Autodesk Fusion 360 part; units mm, degrees
(part 2 of 6)
sketch "Sketch3" plane through (0, 0, 0) normal (0, 1, 0) x (-1, 0, 0)
  line L0 (-39.9203, -22.8327) -> (-39.9203, -25.9319)
  line L1 (-39.9203, -25.9319) -> (-40.7211, -25.9319)
  line L2 (-40.7211, -25.9319) -> (-40.7211, -31.7321)
  line L3 (-40.7211, -31.7321) -> (-39.9203, -31.7321)
  line L4 (-39.9203, -31.7321) -> (-39.9203, -34.8327)
  line L5 (-39.9203, -34.8327) -> (-40.7211, -34.8327)
  line L6 (-40.7211, -34.8327) -> (-40.7211, -35.8316)
  line L7 (-40.7211, -35.8316) -> (-54.7204, -35.8316)
  line L8 (-54.7204, -35.8316) -> (-54.7204, -34.8327)
  line L9 (-54.7204, -34.8327) -> (-55.5212, -34.8327)
  line L10 (-55.5212, -34.8327) -> (-55.5212, -31.7321)
  line L11 (-55.5212, -31.7321) -> (-54.7204, -31.7321)
  line L12 (-54.7204, -31.7321) -> (-54.7204, -25.9319)
  line L13 (-54.7204, -25.9319) -> (-55.5212, -25.9319)
  line L14 (-55.5212, -25.9319) -> (-55.5212, -22.8327)
  line L15 (-55.5212, -22.8327) -> (-54.7204, -22.8327)
  line L16 (-54.7204, -22.8327) -> (-54.7204, -21.8323)
  line L17 (-54.7204, -21.8323) -> (-40.7211, -21.8323)
  line L18 (-40.7211, -21.8323) -> (-40.7211, -22.8327)
  line L19 (-40.7211, -22.8327) -> (-39.9203, -22.8327)
  line L20 (-111.869, -35.8316) -> (-111.869, -34.8327)
  line L21 (-111.869, -34.8327) -> (-112.67, -34.8327)
  line L22 (-112.67, -34.8327) -> (-112.67, -31.7321)
  line L23 (-112.67, -31.7321) -> (-111.869, -31.7321)
  line L24 (-111.869, -31.7321) -> (-111.869, -25.9319)
  line L25 (-111.869, -25.9319) -> (-112.67, -25.9319)
  line L26 (-112.67, -25.9319) -> (-112.67, -22.8327)
  line L27 (-112.67, -22.8327) -> (-111.869, -22.8327)
  line L28 (-111.869, -22.8327) -> (-111.869, -21.8323)
  line L29 (-111.869, -21.8323) -> (-97.8697, -21.8323)
  line L30 (-97.8697, -21.8323) -> (-97.8697, -22.8327)
  line L31 (-97.8697, -22.8327) -> (-97.0703, -22.8327)
  line L32 (-97.0703, -22.8327) -> (-97.0703, -25.9319)
  line L33 (-97.0703, -25.9319) -> (-97.8697, -25.9319)
  line L34 (-97.8697, -25.9319) -> (-97.8697, -31.7321)
  line L35 (-97.8697, -31.7321) -> (-97.0703, -31.7321)
  line L36 (-97.0703, -31.7321) -> (-97.0703, -34.8327)
  line L37 (-97.0703, -34.8327) -> (-97.8697, -34.8327)
  line L38 (-97.8697, -34.8327) -> (-97.8697, -35.8316)
  line L39 (-97.8697, -35.8316) -> (-111.869, -35.8316)
  line L40 (-78.8211, -34.8327) -> (-78.8211, -35.8316)
  line L41 (-78.8211, -35.8316) -> (-92.8204, -35.8316)
  line L42 (-92.8204, -35.8316) -> (-92.8204, -34.8327)
  line L43 (-92.8204, -34.8327) -> (-93.6198, -34.8327)
  line L44 (-93.6198, -34.8327) -> (-93.6198, -31.7321)
  line L45 (-93.6198, -31.7321) -> (-92.8204, -31.7321)
  line L46 (-92.8204, -31.7321) -> (-92.8204, -25.9319)
  line L47 (-92.8204, -25.9319) -> (-93.6198, -25.9319)
  line L48 (-93.6198, -25.9319) -> (-93.6198, -22.8327)
  line L49 (-93.6198, -22.8327) -> (-92.8204, -22.8327)
  line L50 (-92.8204, -22.8327) -> (-92.8204, -21.8323)
  line L51 (-92.8204, -21.8323) -> (-78.8211, -21.8323)
  line L52 (-78.8211, -21.8323) -> (-78.8211, -22.8327)
  line L53 (-78.8211, -22.8327) -> (-78.0203, -22.8327)
  line L54 (-78.0203, -22.8327) -> (-78.0203, -25.9319)
  line L55 (-78.0203, -25.9319) -> (-78.8211, -25.9319)
  line L56 (-78.8211, -25.9319) -> (-78.8211, -31.7321)
  line L57 (-78.8211, -31.7321) -> (-78.0203, -31.7321)
  line L58 (-78.0203, -31.7321) -> (-78.0203, -34.8327)
  line L59 (-78.0203, -34.8327) -> (-78.8211, -34.8327)
  line L60 (-59.7711, -34.8327) -> (-59.7711, -35.8316)
  line L61 (-59.7711, -35.8316) -> (-73.7704, -35.8316)
  line L62 (-73.7704, -35.8316) -> (-73.7704, -34.8327)
  line L63 (-73.7704, -34.8327) -> (-74.5712, -34.8327)
  line L64 (-74.5712, -34.8327) -> (-74.5712, -31.7321)
  line L65 (-74.5712, -31.7321) -> (-73.7704, -31.7321)
  line L66 (-73.7704, -31.7321) -> (-73.7704, -25.9319)
  line L67 (-73.7704, -25.9319) -> (-74.5712, -25.9319)
  line L68 (-74.5712, -25.9319) -> (-74.5712, -22.8327)
  line L69 (-74.5712, -22.8327) -> (-73.7704, -22.8327)
  line L70 (-73.7704, -22.8327) -> (-73.7704, -21.8323)
  line L71 (-73.7704, -21.8323) -> (-59.7711, -21.8323)
  line L72 (-59.7711, -21.8323) -> (-59.7711, -22.8327)
  line L73 (-59.7711, -22.8327) -> (-58.9703, -22.8327)
  line L74 (-58.9703, -22.8327) -> (-58.9703, -25.9319)
  line L75 (-58.9703, -25.9319) -> (-59.7711, -25.9319)
  line L76 (-59.7711, -25.9319) -> (-59.7711, -31.7321)
  line L77 (-59.7711, -31.7321) -> (-58.9703, -31.7321)
  line L78 (-58.9703, -31.7321) -> (-58.9703, -34.8327)
  line L79 (-58.9703, -34.8327) -> (-59.7711, -34.8327)
  line L80 (-188.871, -41.8828) -> (-188.07, -41.8828)
  line L81 (-188.07, -41.8828) -> (-188.07, -40.8824)
  line L82 (-188.07, -40.8824) -> (-174.071, -40.8824)
  line L83 (-174.071, -40.8824) -> (-174.071, -41.8828)
  line L84 (-174.071, -41.8828) -> (-173.27, -41.8828)
  line L85 (-173.27, -41.8828) -> (-173.27, -44.982)
  line L86 (-173.27, -44.982) -> (-174.071, -44.982)
  line L87 (-174.071, -44.982) -> (-174.071, -50.782)
  line L88 (-174.071, -50.782) -> (-173.27, -50.782)
  line L89 (-173.27, -50.782) -> (-173.27, -53.8826)
  line L90 (-173.27, -53.8826) -> (-174.071, -53.8826)
  line L91 (-174.071, -53.8826) -> (-174.071, -54.8816)
  line L92 (-174.071, -54.8816) -> (-188.07, -54.8816)
  line L93 (-188.07, -54.8816) -> (-188.07, -53.8826)
  line L94 (-188.07, -53.8826) -> (-188.871, -53.8826)
  line L95 (-188.871, -53.8826) -> (-188.871, -50.782)
  line L96 (-188.871, -50.782) -> (-188.07, -50.782)
  line L97 (-188.07, -50.782) -> (-188.07, -44.982)
  line L98 (-188.07, -44.982) -> (-188.871, -44.982)
  line L99 (-188.871, -44.982) -> (-188.871, -41.8828)
  line L100 (-35.6704, -34.8327) -> (-36.4712, -34.8327)
  line L101 (-36.4712, -34.8327) -> (-36.4712, -31.7321)
  line L102 (-36.4712, -31.7321) -> (-35.6704, -31.7321)
  line L103 (-35.6704, -31.7321) -> (-35.6704, -25.9319)
  line L104 (-35.6704, -25.9319) -> (-36.4712, -25.9319)
  line L105 (-36.4712, -25.9319) -> (-36.4712, -22.8327)
  line L106 (-36.4712, -22.8327) -> (-35.6704, -22.8327)
  line L107 (-35.6704, -22.8327) -> (-35.6704, -21.8323)
  line L108 (-35.6704, -21.8323) -> (-21.671, -21.8323)
  line L109 (-21.671, -21.8323) -> (-21.671, -22.8327)
  line L110 (-21.671, -22.8327) -> (-20.8704, -22.8327)
  line L111 (-20.8704, -22.8327) -> (-20.8704, -25.9319)
  line L112 (-20.8704, -25.9319) -> (-21.671, -25.9319)
  line L113 (-21.671, -25.9319) -> (-21.671, -31.7321)
  line L114 (-21.671, -31.7321) -> (-20.8704, -31.7321)
  line L115 (-20.8704, -31.7321) -> (-20.8704, -34.8327)
  line L116 (-20.8704, -34.8327) -> (-21.671, -34.8327)
  line L117 (-21.671, -34.8327) -> (-21.671, -35.8316)
  line L118 (-21.671, -35.8316) -> (-35.6704, -35.8316)
  line L119 (-35.6704, -35.8316) -> (-35.6704, -34.8327)
  line L120 (-2.621, -22.8327) -> (-1.8204, -22.8327)
  line L121 (-1.8204, -22.8327) -> (-1.8204, -25.9319)
  line L122 (-1.8204, -25.9319) -> (-2.621, -25.9319)
  line L123 (-2.621, -25.9319) -> (-2.621, -31.7321)
  line L124 (-2.621, -31.7321) -> (-1.8204, -31.7321)
  line L125 (-1.8204, -31.7321) -> (-1.8204, -34.8327)
  line L126 (-1.8204, -34.8327) -> (-2.621, -34.8327)
  line L127 (-2.621, -34.8327) -> (-2.621, -35.8316)
  line L128 (-2.621, -35.8316) -> (-16.6205, -35.8316)
  line L129 (-16.6205, -35.8316) -> (-16.6205, -34.8327)
  line L130 (-16.6205, -34.8327) -> (-17.4212, -34.8327)
  line L131 (-17.4212, -34.8327) -> (-17.4212, -31.7321)
  line L132 (-17.4212, -31.7321) -> (-16.6205, -31.7321)
  line L133 (-16.6205, -31.7321) -> (-16.6205, -25.9319)
  line L134 (-16.6205, -25.9319) -> (-17.4212, -25.9319)
  line L135 (-17.4212, -25.9319) -> (-17.4212, -22.8327)
  line L136 (-17.4212, -22.8327) -> (-16.6205, -22.8327)
  line L137 (-16.6205, -22.8327) -> (-16.6205, -21.8323)
  line L138 (-16.6205, -21.8323) -> (-2.621, -21.8323)
  line L139 (-2.621, -21.8323) -> (-2.621, -22.8327)
  line L140 (-130.92, -41.8828) -> (-130.92, -40.8824)
  line L141 (-130.92, -40.8824) -> (-116.92, -40.8824)
  line L142 (-116.92, -40.8824) -> (-116.92, -41.8828)
  line L143 (-116.92, -41.8828) -> (-116.119, -41.8828)
  line L144 (-116.119, -41.8828) -> (-116.119, -44.982)
  line L145 (-116.119, -44.982) -> (-116.92, -44.982)
  line L146 (-116.92, -44.982) -> (-116.92, -50.782)
  line L147 (-116.92, -50.782) -> (-116.119, -50.782)
  line L148 (-116.119, -50.782) -> (-116.119, -53.8826)
  line L149 (-116.119, -53.8826) -> (-116.92, -53.8826)
  line L150 (-116.92, -53.8826) -> (-116.92, -54.8816)
  line L151 (-116.92, -54.8816) -> (-130.92, -54.8816)
  line L152 (-130.92, -54.8816) -> (-130.92, -53.8826)
  line L153 (-130.92, -53.8826) -> (-131.721, -53.8826)
  line L154 (-131.721, -53.8826) -> (-131.721, -50.782)
  line L155 (-131.721, -50.782) -> (-130.92, -50.782)
  line L156 (-130.92, -50.782) -> (-130.92, -44.982)
  line L157 (-130.92, -44.982) -> (-131.721, -44.982)
  line L158 (-131.721, -44.982) -> (-131.721, -41.8828)
  line L159 (-131.721, -41.8828) -> (-130.92, -41.8828)
  line L160 (-135.17, -50.782) -> (-135.17, -53.8826)
  line L161 (-135.17, -53.8826) -> (-135.971, -53.8826)
  line L162 (-135.971, -53.8826) -> (-135.971, -54.8816)
  line L163 (-135.971, -54.8816) -> (-149.97, -54.8816)
  line L164 (-149.97, -54.8816) -> (-149.97, -53.8826)
  line L165 (-149.97, -53.8826) -> (-150.771, -53.8826)
  line L166 (-150.771, -53.8826) -> (-150.771, -50.782)
  line L167 (-150.771, -50.782) -> (-149.97, -50.782)
  line L168 (-149.97, -50.782) -> (-149.97, -44.982)
  line L169 (-149.97, -44.982) -> (-150.771, -44.982)
  line L170 (-150.771, -44.982) -> (-150.771, -41.8828)
  line L171 (-150.771, -41.8828) -> (-149.97, -41.8828)
  line L172 (-149.97, -41.8828) -> (-149.97, -40.8824)
  line L173 (-149.97, -40.8824) -> (-135.971, -40.8824)
  line L174 (-135.971, -40.8824) -> (-135.971, -41.8828)
  line L175 (-135.971, -41.8828) -> (-135.17, -41.8828)
  line L176 (-135.17, -41.8828) -> (-135.17, -44.982)
  line L177 (-135.17, -44.982) -> (-135.971, -44.982)
  line L178 (-135.971, -44.982) -> (-135.971, -50.782)
  line L179 (-135.971, -50.782) -> (-135.17, -50.782)
  line L180 (-169.821, -53.8826) -> (-169.821, -50.782)
  line L181 (-169.821, -50.782) -> (-169.02, -50.782)
  line L182 (-169.02, -50.782) -> (-169.02, -44.982)
  line L183 (-169.02, -44.982) -> (-169.821, -44.982)
  line L184 (-169.821, -44.982) -> (-169.821, -41.8828)
  line L185 (-169.821, -41.8828) -> (-169.02, -41.8828)
  line L186 (-169.02, -41.8828) -> (-169.02, -40.8824)
  line L187 (-169.02, -40.8824) -> (-155.021, -40.8824)
  line L188 (-155.021, -40.8824) -> (-155.021, -41.8828)
  line L189 (-155.021, -41.8828) -> (-154.22, -41.8828)
  line L190 (-154.22, -41.8828) -> (-154.22, -44.982)
  line L191 (-154.22, -44.982) -> (-155.021, -44.982)
  line L192 (-155.021, -44.982) -> (-155.021, -50.782)
  line L193 (-155.021, -50.782) -> (-154.22, -50.782)
  line L194 (-154.22, -50.782) -> (-154.22, -53.8826)
  line L195 (-154.22, -53.8826) -> (-155.021, -53.8826)
  line L196 (-155.021, -53.8826) -> (-155.021, -54.8816)
  line L197 (-155.021, -54.8816) -> (-169.02, -54.8816)
  line L198 (-169.02, -54.8816) -> (-169.02, -53.8826)
  line L199 (-169.02, -53.8826) -> (-169.821, -53.8826)
  line L200 (-111.869, -44.982) -> (-112.67, -44.982)
  line L201 (-112.67, -44.982) -> (-112.67, -41.8828)
  line L202 (-112.67, -41.8828) -> (-111.869, -41.8828)
  line L203 (-111.869, -41.8828) -> (-111.869, -40.8824)
  line L204 (-111.869, -40.8824) -> (-97.8697, -40.8824)
  line L205 (-97.8697, -40.8824) -> (-97.8697, -41.8828)
  line L206 (-97.8697, -41.8828) -> (-97.0703, -41.8828)
  line L207 (-97.0703, -41.8828) -> (-97.0703, -44.982)
  line L208 (-97.0703, -44.982) -> (-97.8697, -44.982)
  line L209 (-97.8697, -44.982) -> (-97.8697, -50.782)
  line L210 (-97.8697, -50.782) -> (-97.0703, -50.782)
  line L211 (-97.0703, -50.782) -> (-97.0703, -53.8826)
  line L212 (-97.0703, -53.8826) -> (-97.8697, -53.8826)
  line L213 (-97.8697, -53.8826) -> (-97.8697, -54.8816)
  line L214 (-97.8697, -54.8816) -> (-111.869, -54.8816)
  line L215 (-111.869, -54.8816) -> (-111.869, -53.8826)
  line L216 (-111.869, -53.8826) -> (-112.67, -53.8826)
  line L217 (-112.67, -53.8826) -> (-112.67, -50.782)
  line L218 (-112.67, -50.782) -> (-111.869, -50.782)
  line L219 (-111.869, -50.782) -> (-111.869, -44.982)
  line L220 (-93.6198, -41.8828) -> (-92.8204, -41.8828)
  line L221 (-92.8204, -41.8828) -> (-92.8204, -40.8824)
  line L222 (-92.8204, -40.8824) -> (-78.8211, -40.8824)
  line L223 (-78.8211, -40.8824) -> (-78.8211, -41.8828)
  line L224 (-78.8211, -41.8828) -> (-78.0203, -41.8828)
  line L225 (-78.0203, -41.8828) -> (-78.0203, -44.982)
  line L226 (-78.0203, -44.982) -> (-78.8211, -44.982)
  line L227 (-78.8211, -44.982) -> (-78.8211, -50.782)
  line L228 (-78.8211, -50.782) -> (-78.0203, -50.782)
  line L229 (-78.0203, -50.782) -> (-78.0203, -53.8826)
  line L230 (-78.0203, -53.8826) -> (-78.8211, -53.8826)
  line L231 (-78.8211, -53.8826) -> (-78.8211, -54.8816)
  line L232 (-78.8211, -54.8816) -> (-92.8204, -54.8816)
  line L233 (-92.8204, -54.8816) -> (-92.8204, -53.8826)
  line L234 (-92.8204, -53.8826) -> (-93.6198, -53.8826)
  line L235 (-93.6198, -53.8826) -> (-93.6198, -50.782)
  line L236 (-93.6198, -50.782) -> (-92.8204, -50.782)
  line L237 (-92.8204, -50.782) -> (-92.8204, -44.982)
  line L238 (-92.8204, -44.982) -> (-93.6198, -44.982)
  line L239 (-93.6198, -44.982) -> (-93.6198, -41.8828)
  line L240 (-59.7711, -54.8816) -> (-73.7704, -54.8816)
  line L241 (-73.7704, -54.8816) -> (-73.7704, -53.8826)
  line L242 (-73.7704, -53.8826) -> (-74.5712, -53.8826)
  line L243 (-74.5712, -53.8826) -> (-74.5712, -50.782)
  line L244 (-74.5712, -50.782) -> (-73.7704, -50.782)
  line L245 (-73.7704, -50.782) -> (-73.7704, -44.982)
  line L246 (-73.7704, -44.982) -> (-74.5712, -44.982)
  line L247 (-74.5712, -44.982) -> (-74.5712, -41.8828)
  line L248 (-74.5712, -41.8828) -> (-73.7704, -41.8828)
  line L249 (-73.7704, -41.8828) -> (-73.7704, -40.8824)
  line L250 (-73.7704, -40.8824) -> (-59.7711, -40.8824)
  line L251 (-59.7711, -40.8824) -> (-59.7711, -41.8828)
  line L252 (-59.7711, -41.8828) -> (-58.9703, -41.8828)
  line L253 (-58.9703, -41.8828) -> (-58.9703, -44.982)
  line L254 (-58.9703, -44.982) -> (-59.7711, -44.982)
  line L255 (-59.7711, -44.982) -> (-59.7711, -50.782)
  line L256 (-59.7711, -50.782) -> (-58.9703, -50.782)
  line L257 (-58.9703, -50.782) -> (-58.9703, -53.8826)
  line L258 (-58.9703, -53.8826) -> (-59.7711, -53.8826)
  line L259 (-59.7711, -53.8826) -> (-59.7711, -54.8816)
  line L260 (-55.5212, -53.8826) -> (-55.5212, -50.782)
  line L261 (-55.5212, -50.782) -> (-54.7204, -50.782)
  line L262 (-54.7204, -50.782) -> (-54.7204, -44.982)
  line L263 (-54.7204, -44.982) -> (-55.5212, -44.982)
  line L264 (-55.5212, -44.982) -> (-55.5212, -41.8828)
  line L265 (-55.5212, -41.8828) -> (-54.7204, -41.8828)
  line L266 (-54.7204, -41.8828) -> (-54.7204, -40.8824)
  line L267 (-54.7204, -40.8824) -> (-40.7211, -40.8824)
  line L268 (-40.7211, -40.8824) -> (-40.7211, -41.8828)
  line L269 (-40.7211, -41.8828) -> (-39.9203, -41.8828)
  line L270 (-39.9203, -41.8828) -> (-39.9203, -44.982)
  line L271 (-39.9203, -44.982) -> (-40.7211, -44.982)
  line L272 (-40.7211, -44.982) -> (-40.7211, -50.782)
  line L273 (-40.7211, -50.782) -> (-39.9203, -50.782)
  line L274 (-39.9203, -50.782) -> (-39.9203, -53.8826)
  line L275 (-39.9203, -53.8826) -> (-40.7211, -53.8826)
  line L276 (-40.7211, -53.8826) -> (-40.7211, -54.8816)
  line L277 (-40.7211, -54.8816) -> (-54.7204, -54.8816)
  line L278 (-54.7204, -54.8816) -> (-54.7204, -53.8826)
  line L279 (-54.7204, -53.8826) -> (-55.5212, -53.8826)
  line L280 (-2.621, -50.782) -> (-1.8204, -50.782)
  line L281 (-1.8204, -50.782) -> (-1.8204, -53.8826)
  line L282 (-1.8204, -53.8826) -> (-2.621, -53.8826)
  line L283 (-2.621, -53.8826) -> (-2.621, -54.8816)
  line L284 (-2.621, -54.8816) -> (-16.6205, -54.8816)
  line L285 (-16.6205, -54.8816) -> (-16.6205, -53.8826)
  line L286 (-16.6205, -53.8826) -> (-17.4212, -53.8826)
  line L287 (-17.4212, -53.8826) -> (-17.4212, -50.782)
  line L288 (-17.4212, -50.782) -> (-16.6205, -50.782)
  line L289 (-16.6205, -50.782) -> (-16.6205, -44.982)
  line L290 (-16.6205, -44.982) -> (-17.4212, -44.982)
  line L291 (-17.4212, -44.982) -> (-17.4212, -41.8828)
  line L292 (-17.4212, -41.8828) -> (-16.6205, -41.8828)
  line L293 (-16.6205, -41.8828) -> (-16.6205, -40.8824)
  line L294 (-16.6205, -40.8824) -> (-2.621, -40.8824)
  line L295 (-2.621, -40.8824) -> (-2.621, -41.8828)
  line L296 (-2.621, -41.8828) -> (-1.8204, -41.8828)
  line L297 (-1.8204, -41.8828) -> (-1.8204, -44.982)
  line L298 (-1.8204, -44.982) -> (-2.621, -44.982)
  line L299 (-2.621, -44.982) -> (-2.621, -50.782)
  line L300 (-35.6704, -53.8826) -> (-36.4712, -53.8826)
  line L301 (-36.4712, -53.8826) -> (-36.4712, -50.782)
  line L302 (-36.4712, -50.782) -> (-35.6704, -50.782)
  line L303 (-35.6704, -50.782) -> (-35.6704, -44.982)
  line L304 (-35.6704, -44.982) -> (-36.4712, -44.982)
  line L305 (-36.4712, -44.982) -> (-36.4712, -41.8828)
  line L306 (-36.4712, -41.8828) -> (-35.6704, -41.8828)
  line L307 (-35.6704, -41.8828) -> (-35.6704, -40.8824)
  line L308 (-35.6704, -40.8824) -> (-21.671, -40.8824)
  line L309 (-21.671, -40.8824) -> (-21.671, -41.8828)
  line L310 (-21.671, -41.8828) -> (-20.8704, -41.8828)
  line L311 (-20.8704, -41.8828) -> (-20.8704, -44.982)
  line L312 (-20.8704, -44.982) -> (-21.671, -44.982)
  line L313 (-21.671, -44.982) -> (-21.671, -50.782)
  line L314 (-21.671, -50.782) -> (-20.8704, -50.782)
  line L315 (-20.8704, -50.782) -> (-20.8704, -53.8826)
  line L316 (-20.8704, -53.8826) -> (-21.671, -53.8826)
  line L317 (-21.671, -53.8826) -> (-21.671, -54.8816)
  line L318 (-21.671, -54.8816) -> (-35.6704, -54.8816)
  line L319 (-35.6704, -54.8816) -> (-35.6704, -53.8826)
  line L320 (-163.745, -3.7827) -> (-163.745, -6.8819)
  line L321 (-163.745, -6.8819) -> (-164.546, -6.8819)
  line L322 (-164.546, -6.8819) -> (-164.546, -12.6821)
  line L323 (-164.546, -12.6821) -> (-163.745, -12.6821)
  line L324 (-163.745, -12.6821) -> (-163.745, -15.7827)
  line L325 (-163.745, -15.7827) -> (-164.546, -15.7827)
  line L326 (-164.546, -15.7827) -> (-164.546, -16.7817)
  line L327 (-164.546, -16.7817) -> (-178.545, -16.7817)
  line L328 (-178.545, -16.7817) -> (-178.545, -15.7827)
  line L329 (-178.545, -15.7827) -> (-179.346, -15.7827)
  line L330 (-179.346, -15.7827) -> (-179.346, -12.6821)
  line L331 (-179.346, -12.6821) -> (-178.545, -12.6821)
  line L332 (-178.545, -12.6821) -> (-178.545, -6.8819)
  line L333 (-178.545, -6.8819) -> (-179.346, -6.8819)
  line L334 (-179.346, -6.8819) -> (-179.346, -3.7827)
  line L335 (-179.346, -3.7827) -> (-178.545, -3.7827)
  line L336 (-178.545, -3.7827) -> (-178.545, -2.7823)
  line L337 (-178.545, -2.7823) -> (-164.546, -2.7823)
  line L338 (-164.546, -2.7823) -> (-164.546, -3.7827)
  line L339 (-164.546, -3.7827) -> (-163.745, -3.7827)
  line L340 (-120.146, -12.0826) -> (-120.971, -12.0826)
  line L341 (-120.971, -12.0826) -> (-120.971, -9.2825)
  line L342 (-120.971, -9.2825) -> (-120.146, -9.2825)
  line L343 (-120.146, -9.2825) -> (-120.146, -3.0138)
  line L344 (-120.146, -3.0138) -> (-118.42, -3.0138)
  line L345 (-118.42, -3.0138) -> (-118.42, -2.0326)
  line L346 (-118.42, -2.0326) -> (-115.12, -2.0326)
  line L347 (-115.12, -2.0326) -> (-115.12, -3.0138)
  line L348 (-115.12, -3.0138) -> (-113.396, -3.0138)
  line L349 (-113.396, -3.0138) -> (-113.396, -7.4827)
  line L350 (-113.396, -7.4827) -> (-111.87, -7.4827)
  line L351 (-111.87, -7.4827) -> (-111.87, -6.8819)
  line L352 (-111.87, -6.8819) -> (-112.671, -6.8819)
  line L353 (-112.671, -6.8819) -> (-112.671, -3.7827)
  line L354 (-112.671, -3.7827) -> (-111.87, -3.7827)
  line L355 (-111.87, -3.7827) -> (-111.87, -2.7823)
  line L356 (-111.87, -2.7823) -> (-97.8711, -2.7823)
  line L357 (-97.8711, -2.7823) -> (-97.8711, -3.7827)
  line L358 (-97.8711, -3.7827) -> (-97.0703, -3.7827)
  line L359 (-97.0703, -3.7827) -> (-97.0703, -6.8819)
  line L360 (-97.0703, -6.8819) -> (-97.8711, -6.8819)
  line L361 (-97.8711, -6.8819) -> (-97.8711, -7.4827)
  line L362 (-97.8711, -7.4827) -> (-96.3454, -7.4827)
  line L363 (-96.3454, -7.4827) -> (-96.3454, -3.0138)
  line L364 (-96.3454, -3.0138) -> (-94.6203, -3.0138)
  line L365 (-94.6203, -3.0138) -> (-94.6203, -2.0326)
  line L366 (-94.6203, -2.0326) -> (-91.3197, -2.0326)
  line L367 (-91.3197, -2.0326) -> (-91.3197, -3.0138)
  line L368 (-91.3197, -3.0138) -> (-89.596, -3.0138)
  line L369 (-89.596, -3.0138) -> (-89.596, -9.2825)
  line L370 (-89.596, -9.2825) -> (-88.7705, -9.2825)
  line L371 (-88.7705, -9.2825) -> (-88.7705, -12.0826)
  line L372 (-88.7705, -12.0826) -> (-89.596, -12.0826)
  line L373 (-89.596, -12.0826) -> (-89.596, -15.3128)
  line L374 (-89.596, -15.3128) -> (-91.3197, -15.3128)
  line L375 (-91.3197, -15.3128) -> (-91.3197, -16.2319)
  line L376 (-91.3197, -16.2319) -> (-94.6203, -16.2319)
  line L377 (-94.6203, -16.2319) -> (-94.6203, -15.3128)
  line L378 (-94.6203, -15.3128) -> (-96.3454, -15.3128)
  line L379 (-96.3454, -15.3128) -> (-96.3454, -12.0826)
  line L380 (-96.3454, -12.0826) -> (-97.8711, -12.0826)
  line L381 (-97.8711, -12.0826) -> (-97.8711, -12.6821)
  line L382 (-97.8711, -12.6821) -> (-97.0703, -12.6821)
  line L383 (-97.0703, -12.6821) -> (-97.0703, -15.7827)
  line L384 (-97.0703, -15.7827) -> (-97.8711, -15.7827)
  line L385 (-97.8711, -15.7827) -> (-97.8711, -16.7817)
  line L386 (-97.8711, -16.7817) -> (-111.87, -16.7817)
  line L387 (-111.87, -16.7817) -> (-111.87, -15.7827)
  line L388 (-111.87, -15.7827) -> (-112.671, -15.7827)
  line L389 (-112.671, -15.7827) -> (-112.671, -12.6821)
  line L390 (-112.671, -12.6821) -> (-111.87, -12.6821)
  line L391 (-111.87, -12.6821) -> (-111.87, -12.0826)
  line L392 (-111.87, -12.0826) -> (-113.396, -12.0826)
  line L393 (-113.396, -12.0826) -> (-113.396, -15.3128)
  line L394 (-113.396, -15.3128) -> (-115.12, -15.3128)
  line L395 (-115.12, -15.3128) -> (-115.12, -16.2319)
  line L396 (-115.12, -16.2319) -> (-118.42, -16.2319)
  line L397 (-118.42, -16.2319) -> (-118.42, -15.3128)
  line L398 (-118.42, -15.3128) -> (-120.146, -15.3128)
  line L399 (-120.146, -15.3128) -> (-120.146, -12.0826)
  line L400 (-140.445, -3.7827) -> (-140.445, -2.7823)
  line L401 (-140.445, -2.7823) -> (-126.446, -2.7823)
  line L402 (-126.446, -2.7823) -> (-126.446, -3.7827)
  line L403 (-126.446, -3.7827) -> (-125.645, -3.7827)
  line L404 (-125.645, -3.7827) -> (-125.645, -6.8819)
  line L405 (-125.645, -6.8819) -> (-126.446, -6.8819)
  line L406 (-126.446, -6.8819) -> (-126.446, -12.6821)
  line L407 (-126.446, -12.6821) -> (-125.645, -12.6821)
  line L408 (-125.645, -12.6821) -> (-125.645, -15.7827)
  line L409 (-125.645, -15.7827) -> (-126.446, -15.7827)
  line L410 (-126.446, -15.7827) -> (-126.446, -16.7817)
  line L411 (-126.446, -16.7817) -> (-140.445, -16.7817)
  line L412 (-140.445, -16.7817) -> (-140.445, -15.7827)
  line L413 (-140.445, -15.7827) -> (-141.246, -15.7827)
  line L414 (-141.246, -15.7827) -> (-141.246, -12.6821)
  line L415 (-141.246, -12.6821) -> (-140.445, -12.6821)
  line L416 (-140.445, -12.6821) -> (-140.445, -6.8819)
  line L417 (-140.445, -6.8819) -> (-141.246, -6.8819)
  line L418 (-141.246, -6.8819) -> (-141.246, -3.7827)
  line L419 (-141.246, -3.7827) -> (-140.445, -3.7827)
  line L420 (-83.2954, -2.7823) -> (-69.2961, -2.7823)
  line L421 (-69.2961, -2.7823) -> (-69.2961, -3.7827)
  line L422 (-69.2961, -3.7827) -> (-68.4953, -3.7827)
  line L423 (-68.4953, -3.7827) -> (-68.4953, -6.8819)
  line L424 (-68.4953, -6.8819) -> (-69.2961, -6.8819)
  line L425 (-69.2961, -6.8819) -> (-69.2961, -12.6821)
  line L426 (-69.2961, -12.6821) -> (-68.4953, -12.6821)
  line L427 (-68.4953, -12.6821) -> (-68.4953, -15.7827)
  line L428 (-68.4953, -15.7827) -> (-69.2961, -15.7827)
  line L429 (-69.2961, -15.7827) -> (-69.2961, -16.7817)
  line L430 (-69.2961, -16.7817) -> (-83.2954, -16.7817)
  line L431 (-83.2954, -16.7817) -> (-83.2954, -15.7827)
  line L432 (-83.2954, -15.7827) -> (-84.0962, -15.7827)
  line L433 (-84.0962, -15.7827) -> (-84.0962, -12.6821)
  line L434 (-84.0962, -12.6821) -> (-83.2954, -12.6821)
  line L435 (-83.2954, -12.6821) -> (-83.2954, -6.8819)
  line L436 (-83.2954, -6.8819) -> (-84.0962, -6.8819)
  line L437 (-84.0962, -6.8819) -> (-84.0962, -3.7827)
  line L438 (-84.0962, -3.7827) -> (-83.2954, -3.7827)
  line L439 (-83.2954, -3.7827) -> (-83.2954, -2.7823)
  line L440 (-64.2454, -16.7817) -> (-64.2454, -15.7827)
  line L441 (-64.2454, -15.7827) -> (-65.0462, -15.7827)
  line L442 (-65.0462, -15.7827) -> (-65.0462, -12.6821)
  line L443 (-65.0462, -12.6821) -> (-64.2454, -12.6821)
  line L444 (-64.2454, -12.6821) -> (-64.2454, -6.8819)
  line L445 (-64.2454, -6.8819) -> (-65.0462, -6.8819)
  line L446 (-65.0462, -6.8819) -> (-65.0462, -3.7827)
  line L447 (-65.0462, -3.7827) -> (-64.2454, -3.7827)
  line L448 (-64.2454, -3.7827) -> (-64.2454, -2.7823)
  line L449 (-64.2454, -2.7823) -> (-50.2461, -2.7823)
  line L450 (-50.2461, -2.7823) -> (-50.2461, -3.7827)
  line L451 (-50.2461, -3.7827) -> (-49.4453, -3.7827)
  line L452 (-49.4453, -3.7827) -> (-49.4453, -6.8819)
  line L453 (-49.4453, -6.8819) -> (-50.2461, -6.8819)
  line L454 (-50.2461, -6.8819) -> (-50.2461, -12.6821)
  line L455 (-50.2461, -12.6821) -> (-49.4453, -12.6821)
  line L456 (-49.4453, -12.6821) -> (-49.4453, -15.7827)
  line L457 (-49.4453, -15.7827) -> (-50.2461, -15.7827)
  line L458 (-50.2461, -15.7827) -> (-50.2461, -16.7817)
  line L459 (-50.2461, -16.7817) -> (-64.2454, -16.7817)
  line L460 (-45.1954, -6.8819) -> (-45.9962, -6.8819)
  line L461 (-45.9962, -6.8819) -> (-45.9962, -3.7827)
  line L462 (-45.9962, -3.7827) -> (-45.1954, -3.7827)
  line L463 (-45.1954, -3.7827) -> (-45.1954, -2.7823)
  line L464 (-45.1954, -2.7823) -> (-31.196, -2.7823)
  line L465 (-31.196, -2.7823) -> (-31.196, -3.7827)
  line L466 (-31.196, -3.7827) -> (-30.3954, -3.7827)
  line L467 (-30.3954, -3.7827) -> (-30.3954, -6.8819)
  line L468 (-30.3954, -6.8819) -> (-31.196, -6.8819)
  line L469 (-31.196, -6.8819) -> (-31.196, -12.6821)
  line L470 (-31.196, -12.6821) -> (-30.3954, -12.6821)
  line L471 (-30.3954, -12.6821) -> (-30.3954, -15.7827)
  line L472 (-30.3954, -15.7827) -> (-31.196, -15.7827)
  line L473 (-31.196, -15.7827) -> (-31.196, -16.7817)
  line L474 (-31.196, -16.7817) -> (-45.1954, -16.7817)
  line L475 (-45.1954, -16.7817) -> (-45.1954, -15.7827)
  line L476 (-45.1954, -15.7827) -> (-45.9962, -15.7827)
  line L477 (-45.9962, -15.7827) -> (-45.9962, -12.6821)
  line L478 (-45.9962, -12.6821) -> (-45.1954, -12.6821)
  line L479 (-45.1954, -12.6821) -> (-45.1954, -6.8819)
  line L480 (-159.495, -6.8819) -> (-160.296, -6.8819)
  line L481 (-160.296, -6.8819) -> (-160.296, -3.7827)
  line L482 (-160.296, -3.7827) -> (-159.495, -3.7827)
  line L483 (-159.495, -3.7827) -> (-159.495, -2.7823)
  line L484 (-159.495, -2.7823) -> (-145.496, -2.7823)
  line L485 (-145.496, -2.7823) -> (-145.496, -3.7827)
  line L486 (-145.496, -3.7827) -> (-144.695, -3.7827)
  line L487 (-144.695, -3.7827) -> (-144.695, -6.8819)
  line L488 (-144.695, -6.8819) -> (-145.496, -6.8819)
  line L489 (-145.496, -6.8819) -> (-145.496, -12.6821)
  line L490 (-145.496, -12.6821) -> (-144.695, -12.6821)
  line L491 (-144.695, -12.6821) -> (-144.695, -15.7827)
  line L492 (-144.695, -15.7827) -> (-145.496, -15.7827)
  line L493 (-145.496, -15.7827) -> (-145.496, -16.7817)
  line L494 (-145.496, -16.7817) -> (-159.495, -16.7817)
  line L495 (-159.495, -16.7817) -> (-159.495, -15.7827)
  line L496 (-159.495, -15.7827) -> (-160.296, -15.7827)
  line L497 (-160.296, -15.7827) -> (-160.296, -12.6821)
  line L498 (-160.296, -12.6821) -> (-159.495, -12.6821)
  line L499 (-159.495, -12.6821) -> (-159.495, -6.8819)
  line L500 (-12.146, -12.6821) -> (-11.3454, -12.6821)
  line L501 (-11.3454, -12.6821) -> (-11.3454, -15.7827)
  line L502 (-11.3454, -15.7827) -> (-12.146, -15.7827)
  line L503 (-12.146, -15.7827) -> (-12.146, -16.7817)
  line L504 (-12.146, -16.7817) -> (-26.1455, -16.7817)
  line L505 (-26.1455, -16.7817) -> (-26.1455, -15.7827)
  line L506 (-26.1455, -15.7827) -> (-26.9462, -15.7827)
  line L507 (-26.9462, -15.7827) -> (-26.9462, -12.6821)
  line L508 (-26.9462, -12.6821) -> (-26.1455, -12.6821)
  line L509 (-26.1455, -12.6821) -> (-26.1455, -6.8819)
  line L510 (-26.1455, -6.8819) -> (-26.9462, -6.8819)
  line L511 (-26.9462, -6.8819) -> (-26.9462, -3.7827)
  line L512 (-26.9462, -3.7827) -> (-26.1455, -3.7827)
  line L513 (-26.1455, -3.7827) -> (-26.1455, -2.7823)
  line L514 (-26.1455, -2.7823) -> (-12.146, -2.7823)
  line L515 (-12.146, -2.7823) -> (-12.146, -3.7827)
  line L516 (-12.146, -3.7827) -> (-11.3454, -3.7827)
  line L517 (-11.3454, -3.7827) -> (-11.3454, -6.8819)
  line L518 (-11.3454, -6.8819) -> (-12.146, -6.8819)
  line L519 (-12.146, -6.8819) -> (-12.146, -12.6821)
  line L520 (-116.119, -25.9319) -> (-116.92, -25.9319)
  line L521 (-116.92, -25.9319) -> (-116.92, -31.7321)
  line L522 (-116.92, -31.7321) -> (-116.119, -31.7321)
  line L523 (-116.119, -31.7321) -> (-116.119, -34.8327)
  line L524 (-116.119, -34.8327) -> (-116.92, -34.8327)
  line L525 (-116.92, -34.8327) -> (-116.92, -35.8316)
  line L526 (-116.92, -35.8316) -> (-130.92, -35.8316)
  line L527 (-130.92, -35.8316) -> (-130.92, -34.8327)
  line L528 (-130.92, -34.8327) -> (-131.721, -34.8327)
  line L529 (-131.721, -34.8327) -> (-131.721, -31.7321)
  line L530 (-131.721, -31.7321) -> (-130.92, -31.7321)
  line L531 (-130.92, -31.7321) -> (-130.92, -25.9319)
  line L532 (-130.92, -25.9319) -> (-131.721, -25.9319)
  line L533 (-131.721, -25.9319) -> (-131.721, -22.8327)
  line L534 (-131.721, -22.8327) -> (-130.92, -22.8327)
  line L535 (-130.92, -22.8327) -> (-130.92, -21.8323)
  line L536 (-130.92, -21.8323) -> (-116.92, -21.8323)
  line L537 (-116.92, -21.8323) -> (-116.92, -22.8327)
  line L538 (-116.92, -22.8327) -> (-116.119, -22.8327)
  line L539 (-116.119, -22.8327) -> (-116.119, -25.9319)
  line L540 (-169.02, -31.7321) -> (-169.02, -25.9319)
  line L541 (-169.02, -25.9319) -> (-169.821, -25.9319)
  line L542 (-169.821, -25.9319) -> (-169.821, -22.8327)
  line L543 (-169.821, -22.8327) -> (-169.02, -22.8327)
  line L544 (-169.02, -22.8327) -> (-169.02, -21.8323)
  line L545 (-169.02, -21.8323) -> (-155.021, -21.8323)
  line L546 (-155.021, -21.8323) -> (-155.021, -22.8327)
  line L547 (-155.021, -22.8327) -> (-154.22, -22.8327)
  line L548 (-154.22, -22.8327) -> (-154.22, -25.9319)
  line L549 (-154.22, -25.9319) -> (-155.021, -25.9319)
  line L550 (-155.021, -25.9319) -> (-155.021, -31.7321)
  line L551 (-155.021, -31.7321) -> (-154.22, -31.7321)
  line L552 (-154.22, -31.7321) -> (-154.22, -34.8327)
  line L553 (-154.22, -34.8327) -> (-155.021, -34.8327)
  line L554 (-155.021, -34.8327) -> (-155.021, -35.8316)
  line L555 (-155.021, -35.8316) -> (-169.02, -35.8316)
  line L556 (-169.02, -35.8316) -> (-169.02, -34.8327)
  line L557 (-169.02, -34.8327) -> (-169.821, -34.8327)
  line L558 (-169.821, -34.8327) -> (-169.821, -31.7321)
  line L559 (-169.821, -31.7321) -> (-169.02, -31.7321)
  line L560 (-135.17, -34.8327) -> (-135.971, -34.8327)
  line L561 (-135.971, -34.8327) -> (-135.971, -35.8316)
  line L562 (-135.971, -35.8316) -> (-149.97, -35.8316)
  line L563 (-149.97, -35.8316) -> (-149.97, -34.8327)
  line L564 (-149.97, -34.8327) -> (-150.771, -34.8327)
  line L565 (-150.771, -34.8327) -> (-150.771, -31.7321)
  line L566 (-150.771, -31.7321) -> (-149.97, -31.7321)
  line L567 (-149.97, -31.7321) -> (-149.97, -25.9319)
  line L568 (-149.97, -25.9319) -> (-150.771, -25.9319)
  line L569 (-150.771, -25.9319) -> (-150.771, -22.8327)
  line L570 (-150.771, -22.8327) -> (-149.97, -22.8327)
  line L571 (-149.97, -22.8327) -> (-149.97, -21.8323)
  line L572 (-149.97, -21.8323) -> (-135.971, -21.8323)
  line L573 (-135.971, -21.8323) -> (-135.971, -22.8327)
  line L574 (-135.971, -22.8327) -> (-135.17, -22.8327)
  line L575 (-135.17, -22.8327) -> (-135.17, -25.9319)
  line L576 (-135.17, -25.9319) -> (-135.971, -25.9319)
  line L577 (-135.971, -25.9319) -> (-135.971, -31.7321)
  line L578 (-135.971, -31.7321) -> (-135.17, -31.7321)
  line L579 (-135.17, -31.7321) -> (-135.17, -34.8327)
  line L580 (-173.27, -25.9319) -> (-174.071, -25.9319)
  line L581 (-174.071, -25.9319) -> (-174.071, -31.7321)
  line L582 (-174.071, -31.7321) -> (-173.27, -31.7321)
  line L583 (-173.27, -31.7321) -> (-173.27, -34.8327)
  line L584 (-173.27, -34.8327) -> (-174.071, -34.8327)
  line L585 (-174.071, -34.8327) -> (-174.071, -35.8316)
  line L586 (-174.071, -35.8316) -> (-188.07, -35.8316)
  line L587 (-188.07, -35.8316) -> (-188.07, -34.8327)
  line L588 (-188.07, -34.8327) -> (-188.871, -34.8327)
  line L589 (-188.871, -34.8327) -> (-188.871, -31.7321)
  line L590 (-188.871, -31.7321) -> (-188.07, -31.7321)
  line L591 (-188.07, -31.7321) -> (-188.07, -25.9319)
  line L592 (-188.07, -25.9319) -> (-188.871, -25.9319)
  line L593 (-188.871, -25.9319) -> (-188.871, -22.8327)
  line L594 (-188.871, -22.8327) -> (-188.07, -22.8327)
  line L595 (-188.07, -22.8327) -> (-188.07, -21.8323)
  line L596 (-188.07, -21.8323) -> (-174.071, -21.8323)
  line L597 (-174.071, -21.8323) -> (-174.071, -22.8327)
  line L598 (-174.071, -22.8327) -> (-173.27, -22.8327)
  line L599 (-173.27, -22.8327) -> (-173.27, -25.9319)
  line L600 (-0.102, -55.5639) -> (-0.0951, -55.4069)
  line L601 (-0.0951, -55.4069) -> (-0.0951, -2.2572)
  line L602 (-0.0951, -2.2572) -> (-0.102, -2.1001)
  line L603 (-0.102, -2.1001) -> (-0.1199, -1.9444)
  line L604 (-0.1199, -1.9444) -> (-0.1502, -1.7901)
  line L605 (-0.1502, -1.7901) -> (-0.1929, -1.6385)
  line L606 (-0.1929, -1.6385) -> (-0.248, -1.491)
  line L607 (-0.248, -1.491) -> (-0.3128, -1.3491)
  line L608 (-0.3128, -1.3491) -> (-0.39, -1.2127)
  line L609 (-0.39, -1.2127) -> (-0.4768, -1.0818)
  line L610 (-0.4768, -1.0818) -> (-0.5746, -0.9577)
  line L611 (-0.5746, -0.9577) -> (-0.6808, -0.842)
  line L612 (-0.6808, -0.842) -> (-0.7965, -0.7359)
  line L613 (-0.7965, -0.7359) -> (-0.9192, -0.638)
  line L614 (-0.9192, -0.638) -> (-1.0501, -0.5512)
  line L615 (-1.0501, -0.5512) -> (-1.1879, -0.474)
  line L616 (-1.1879, -0.474) -> (-1.3298, -0.4093)
  line L617 (-1.3298, -0.4093) -> (-1.4759, -0.3542)
  line L618 (-1.4759, -0.3542) -> (-1.6288, -0.3128)
  line L619 (-1.6288, -0.3128) -> (-1.7818, -0.2811)
  line L620 (-1.7818, -0.2811) -> (-1.9389, -0.2632)
  line L621 (-1.9389, -0.2632) -> (-2.096, -0.2577)
  line L622 (-2.096, -0.2577) -> (-23.4739, -0.2575)
  line L623 (-188.597, -0.2563) -> (-188.753, -0.2632)
  line L624 (-188.753, -0.2632) -> (-188.908, -0.2811)
  line L625 (-188.908, -0.2811) -> (-189.063, -0.3128)
  line L626 (-189.063, -0.3128) -> (-189.214, -0.3542)
  line L627 (-189.214, -0.3542) -> (-189.362, -0.4093)
  line L628 (-189.362, -0.4093) -> (-189.504, -0.474)
  line L629 (-189.504, -0.474) -> (-189.64, -0.5512)
  line L630 (-189.64, -0.5512) -> (-189.771, -0.638)
  line L631 (-189.771, -0.638) -> (-189.895, -0.7359)
  line L632 (-189.895, -0.7359) -> (-190.011, -0.842)
  line L633 (-190.011, -0.842) -> (-190.117, -0.9577)
  line L634 (-190.117, -0.9577) -> (-190.215, -1.0818)
  line L635 (-190.215, -1.0818) -> (-190.302, -1.2127)
  line L636 (-190.302, -1.2127) -> (-190.379, -1.3491)
  line L637 (-190.379, -1.3491) -> (-190.444, -1.491)
  line L638 (-190.444, -1.491) -> (-190.499, -1.6385)
  line L639 (-190.499, -1.6385) -> (-190.54, -1.7901)
  line L640 (-190.54, -1.7901) -> (-190.572, -1.9444)
  line L641 (-190.572, -1.9444) -> (-190.59, -2.1001)
  line L642 (-190.59, -2.1001) -> (-190.596, -2.2572)
  line L643 (-190.596, -2.2572) -> (-190.596, -55.4069)
  line L644 (-190.596, -55.4069) -> (-190.59, -55.5639)
  line L645 (-190.59, -55.5639) -> (-190.572, -55.7209)
  line L646 (-190.572, -55.7209) -> (-190.54, -55.874)
  line L647 (-190.54, -55.874) -> (-190.499, -56.0268)
  line L648 (-190.499, -56.0268) -> (-190.444, -56.1728)
  line L649 (-190.444, -56.1728) -> (-190.379, -56.315)
  line L650 (-190.379, -56.315) -> (-190.302, -56.4526)
  line L651 (-190.302, -56.4526) -> (-190.215, -56.5838)
  line L652 (-190.215, -56.5838) -> (-190.117, -56.7062)
  line L653 (-190.117, -56.7062) -> (-190.011, -56.8219)
  line L654 (-190.011, -56.8219) -> (-189.895, -56.9281)
  line L655 (-189.895, -56.9281) -> (-189.771, -57.0258)
  line L656 (-189.771, -57.0258) -> (-189.64, -57.113)
  line L657 (-189.64, -57.113) -> (-189.504, -57.1899)
  line L658 (-189.504, -57.1899) -> (-189.362, -57.2548)
  line L659 (-189.362, -57.2548) -> (-189.214, -57.3098)
  line L660 (-189.214, -57.3098) -> (-189.063, -57.3525)
  line L661 (-189.063, -57.3525) -> (-188.908, -57.3828)
  line L662 (-188.908, -57.3828) -> (-188.753, -57.4008)
  line L663 (-188.753, -57.4008) -> (-188.597, -57.4075)
  line L664 (-188.597, -57.4075) -> (-184.1714, -57.4075)
  line L665 (-6.5216, -57.4075) -> (-2.096, -57.4075)
  line L666 (-2.096, -57.4075) -> (-1.9389, -57.4008)
  line L667 (-1.9389, -57.4008) -> (-1.7818, -57.3828)
  line L668 (-1.7818, -57.3828) -> (-1.6288, -57.3525)
  line L669 (-1.6288, -57.3525) -> (-1.4759, -57.3098)
  line L670 (-1.4759, -57.3098) -> (-1.3298, -57.2548)
  line L671 (-1.3298, -57.2548) -> (-1.1879, -57.1899)
  line L672 (-1.1879, -57.1899) -> (-1.0501, -57.113)
  line L673 (-1.0501, -57.113) -> (-0.9192, -57.0258)
  line L674 (-0.9192, -57.0258) -> (-0.7965, -56.9281)
  line L675 (-0.7965, -56.9281) -> (-0.6808, -56.8219)
  line L676 (-0.6808, -56.8219) -> (-0.5746, -56.7062)
  line L677 (-0.5746, -56.7062) -> (-0.4768, -56.5838)
  line L678 (-0.4768, -56.5838) -> (-0.39, -56.4526)
  line L679 (-0.39, -56.4526) -> (-0.3128, -56.315)
  line L680 (-0.3128, -56.315) -> (-0.248, -56.1728)
  line L681 (-0.248, -56.1728) -> (-0.1929, -56.0268)
  line L682 (-0.1929, -56.0268) -> (-0.1502, -55.874)
  line L683 (-0.1502, -55.874) -> (-0.1199, -55.7209)
  line L684 (-0.1199, -55.7209) -> (-0.102, -55.5639)
  line L685 (-12.146, -16.7817) -> (-178.545, -16.7817)
  line L686 (-178.545, -16.7817) -> (-178.545, -17.7817)
  line L687 (-178.545, -17.7817) -> (-12.146, -17.7817)
  line L688 (-12.146, -17.7817) -> (-12.146, -16.7817)
  line L689 (-178.545, -2.7823) -> (-12.146, -2.7823)
  line L690 (-12.146, -2.7823) -> (-12.146, -1.7823)
  line L691 (-12.146, -1.7823) -> (-178.545, -1.7823)
  line L692 (-178.545, -1.7823) -> (-178.545, -2.7823)
  line L693 (-26.1455, -16.7817) -> (-31.196, -16.7817)
  line L694 (-31.196, -16.7817) -> (-31.196, -17.7817)
  line L695 (-31.196, -17.7817) -> (-26.1455, -17.7817)
  line L696 (-26.1455, -17.7817) -> (-26.1455, -16.7817)
  line L697 (-26.1455, -17.7817) -> (-31.196, -17.7817)
  line L698 (-31.196, -17.7817) -> (-31.196, -1.7823)
  line L699 (-31.196, -1.7823) -> (-26.1455, -1.7823)
  line L700 (-26.1455, -1.7823) -> (-26.1455, -17.7817)
  line L701 (-45.1954, -16.7817) -> (-50.2461, -16.7817)
  line L702 (-50.2461, -16.7817) -> (-50.2461, -17.7817)
  line L703 (-50.2461, -17.7817) -> (-45.1954, -17.7817)
  line L704 (-45.1954, -17.7817) -> (-45.1954, -16.7817)
  line L705 (-50.2461, -17.7817) -> (-45.1954, -17.7817)
  line L706 (-45.1954, -17.7817) -> (-45.1954, -1.7823)
  line L707 (-45.1954, -1.7823) -> (-50.2461, -1.7823)
  line L708 (-50.2461, -1.7823) -> (-50.2461, -17.7817)
  line L709 (-64.2454, -16.7817) -> (-69.2961, -16.7817)
  line L710 (-69.2961, -16.7817) -> (-69.2961, -17.7817)
  line L711 (-69.2961, -17.7817) -> (-64.2454, -17.7817)
  line L712 (-64.2454, -17.7817) -> (-64.2454, -16.7817)
  line L713 (-64.2454, -17.7817) -> (-69.2961, -17.7817)
  line L714 (-69.2961, -17.7817) -> (-69.2961, -1.7823)
  line L715 (-69.2961, -1.7823) -> (-64.2454, -1.7823)
  line L716 (-64.2454, -1.7823) -> (-64.2454, -17.7817)
  line L717 (-83.2954, -16.7817) -> (-97.8711, -16.7817)
  line L718 (-97.8711, -16.7817) -> (-97.8711, -17.7817)
  line L719 (-97.8711, -17.7817) -> (-83.2954, -17.7817)
  line L720 (-83.2954, -17.7817) -> (-83.2954, -16.7817)
  line L721 (-83.2954, -2.7823) -> (-97.8711, -2.7823)
  line L722 (-97.8711, -2.7823) -> (-97.8711, -1.7823)
  line L723 (-97.8711, -1.7823) -> (-83.2954, -1.7823)
  line L724 (-83.2954, -1.7823) -> (-83.2954, -2.7823)
  line L725 (-126.446, -16.7817) -> (-111.87, -16.7817)
  line L726 (-111.87, -16.7817) -> (-111.87, -17.7817)
  line L727 (-111.87, -17.7817) -> (-126.446, -17.7817)
  line L728 (-126.446, -17.7817) -> (-126.446, -16.7817)
  line L729 (-111.87, -2.7823) -> (-126.446, -2.7823)
  line L730 (-126.446, -2.7823) -> (-126.446, -1.7823)
  line L731 (-126.446, -1.7823) -> (-111.87, -1.7823)
  line L732 (-111.87, -1.7823) -> (-111.87, -2.7823)
  line L733 (-140.445, -2.7823) -> (-145.496, -2.7823)
  line L734 (-145.496, -2.7823) -> (-145.496, -1.7823)
  line L735 (-145.496, -1.7823) -> (-140.445, -1.7823)
  line L736 (-140.445, -1.7823) -> (-140.445, -2.7823)
  line L737 (-140.445, -16.7817) -> (-145.496, -16.7817)
  line L738 (-145.496, -16.7817) -> (-145.496, -17.7817)
  line L739 (-145.496, -17.7817) -> (-140.445, -17.7817)
  line L740 (-140.445, -17.7817) -> (-140.445, -16.7817)
  line L741 (-159.495, -16.7817) -> (-164.546, -16.7817)
  line L742 (-164.546, -16.7817) -> (-164.546, -17.7817)
  line L743 (-164.546, -17.7817) -> (-159.495, -17.7817)
  line L744 (-159.495, -17.7817) -> (-159.495, -16.7817)
  line L745 (-159.495, -2.7823) -> (-164.546, -2.7823)
  line L746 (-164.546, -2.7823) -> (-164.546, -1.7823)
  line L747 (-164.546, -1.7823) -> (-159.495, -1.7823)
  line L748 (-159.495, -1.7823) -> (-159.495, -2.7823)
  line L749 (-188.07, -35.8316) -> (-2.621, -35.8316)
  line L750 (-2.621, -35.8316) -> (-2.621, -36.8316)
  line L751 (-2.621, -36.8316) -> (-188.07, -36.8316)
  line L752 (-188.07, -36.8316) -> (-188.07, -35.8316)
  line L753 (-2.621, -21.8323) -> (-188.07, -21.8323)
  line L754 (-188.07, -21.8323) -> (-188.07, -20.8323)
  line L755 (-188.07, -20.8323) -> (-2.621, -20.8323)
  line L756 (-2.621, -20.8323) -> (-2.621, -21.8323)
  line L757 (-188.07, -40.8824) -> (-2.621, -40.8824)
  line L758 (-2.621, -40.8824) -> (-2.621, -39.8824)
  line L759 (-2.621, -39.8824) -> (-188.07, -39.8824)
  line L760 (-188.07, -39.8824) -> (-188.07, -40.8824)
  line L761 (-2.621, -54.8816) -> (-188.07, -54.8816)
  line L762 (-188.07, -54.8816) -> (-188.07, -55.8816)
  line L763 (-188.07, -55.8816) -> (-2.621, -55.8816)
  line L764 (-2.621, -55.8816) -> (-2.621, -54.8816)
  line L765 (-174.071, -54.8816) -> (-169.02, -54.8816)
  line L766 (-169.02, -54.8816) -> (-169.02, -55.8816)
  line L767 (-169.02, -55.8816) -> (-174.071, -55.8816)
  line L768 (-174.071, -55.8816) -> (-174.071, -54.8816)
  line L769 (-169.02, -55.8816) -> (-174.071, -55.8816)
  line L770 (-174.071, -55.8816) -> (-174.071, -20.8323)
  line L771 (-174.071, -20.8323) -> (-169.02, -20.8323)
  line L772 (-169.02, -20.8323) -> (-169.02, -55.8816)
  line L773 (-149.97, -21.8323) -> (-155.021, -21.8323)
  line L774 (-155.021, -21.8323) -> (-155.021, -20.8323)
  line L775 (-155.021, -20.8323) -> (-149.97, -20.8323)
  line L776 (-149.97, -20.8323) -> (-149.97, -21.8323)
  line L777 (-155.021, -20.8323) -> (-149.97, -20.8323)
  line L778 (-149.97, -20.8323) -> (-149.97, -55.8816)
  line L779 (-149.97, -55.8816) -> (-155.021, -55.8816)
  line L780 (-155.021, -55.8816) -> (-155.021, -20.8323)
  line L781 (-135.971, -54.8816) -> (-130.92, -54.8816)
  line L782 (-130.92, -54.8816) -> (-130.92, -55.8816)
  line L783 (-130.92, -55.8816) -> (-135.971, -55.8816)
  line L784 (-135.971, -55.8816) -> (-135.971, -54.8816)
  line L785 (-130.92, -55.8816) -> (-135.971, -55.8816)
  line L786 (-135.971, -55.8816) -> (-135.971, -20.8323)
  line L787 (-135.971, -20.8323) -> (-130.92, -20.8323)
  line L788 (-130.92, -20.8323) -> (-130.92, -55.8816)
  line L789 (-116.92, -21.8323) -> (-111.869, -21.8323)
  line L790 (-111.869, -21.8323) -> (-111.869, -20.8323)
  line L791 (-111.869, -20.8323) -> (-116.92, -20.8323)
  line L792 (-116.92, -20.8323) -> (-116.92, -21.8323)
  line L793 (-111.869, -20.8323) -> (-116.92, -20.8323)
  line L794 (-116.92, -20.8323) -> (-116.92, -55.8816)
  line L795 (-116.92, -55.8816) -> (-111.869, -55.8816)
  line L796 (-111.869, -55.8816) -> (-111.869, -20.8323)
  line L797 (-97.8697, -54.8816) -> (-92.8204, -54.8816)
  line L798 (-92.8204, -54.8816) -> (-92.8204, -55.8816)
  line L799 (-92.8204, -55.8816) -> (-97.8697, -55.8816)
  line L800 (-97.8697, -55.8816) -> (-97.8697, -54.8816)
  line L801 (-92.8204, -55.8816) -> (-97.8697, -55.8816)
  line L802 (-97.8697, -55.8816) -> (-97.8697, -20.8323)
  line L803 (-97.8697, -20.8323) -> (-92.8204, -20.8323)
  line L804 (-92.8204, -20.8323) -> (-92.8204, -55.8816)
  line L805 (-78.8211, -21.8323) -> (-73.7704, -21.8323)
  line L806 (-73.7704, -21.8323) -> (-73.7704, -20.8323)
  line L807 (-73.7704, -20.8323) -> (-78.8211, -20.8323)
  line L808 (-78.8211, -20.8323) -> (-78.8211, -21.8323)
  line L809 (-73.7704, -20.8323) -> (-78.8211, -20.8323)
  line L810 (-78.8211, -20.8323) -> (-78.8211, -55.8816)
  line L811 (-78.8211, -55.8816) -> (-73.7704, -55.8816)
  line L812 (-73.7704, -55.8816) -> (-73.7704, -20.8323)
  line L813 (-59.7711, -54.8816) -> (-54.7204, -54.8816)
  line L814 (-54.7204, -54.8816) -> (-54.7204, -55.8816)
  line L815 (-54.7204, -55.8816) -> (-59.7711, -55.8816)
  line L816 (-59.7711, -55.8816) -> (-59.7711, -54.8816)
  line L817 (-54.7204, -55.8816) -> (-59.7711, -55.8816)
  line L818 (-59.7711, -55.8816) -> (-59.7711, -20.8323)
  line L819 (-59.7711, -20.8323) -> (-54.7204, -20.8323)
  line L820 (-54.7204, -20.8323) -> (-54.7204, -55.8816)
  line L821 (-40.7211, -21.8323) -> (-35.6704, -21.8323)
  line L822 (-35.6704, -21.8323) -> (-35.6704, -20.8323)
  line L823 (-35.6704, -20.8323) -> (-40.7211, -20.8323)
  line L824 (-40.7211, -20.8323) -> (-40.7211, -21.8323)
  line L825 (-35.6704, -20.8323) -> (-40.7211, -20.8323)
  line L826 (-40.7211, -20.8323) -> (-40.7211, -55.8816)
  line L827 (-40.7211, -55.8816) -> (-35.6704, -55.8816)
  line L828 (-35.6704, -55.8816) -> (-35.6704, -20.8323)
  line L829 (-21.671, -54.8816) -> (-16.6205, -54.8816)
  line L830 (-16.6205, -54.8816) -> (-16.6205, -55.8816)
  line L831 (-16.6205, -55.8816) -> (-21.671, -55.8816)
  line L832 (-21.671, -55.8816) -> (-21.671, -54.8816)
  line L833 (-16.6205, -55.8816) -> (-21.671, -55.8816)
  line L834 (-21.671, -55.8816) -> (-21.671, -20.8323)
  line L835 (-21.671, -20.8323) -> (-16.6205, -20.8323)
  line L836 (-16.6205, -20.8323) -> (-16.6205, -55.8816)
  spline S0 degree 2 poles (-184.1714, -57.4075) (-176.3801, -57.4075) (-176.3801, -64.9763) knots 0 0 0 1 1 1
  arc A0 (-176.3801, -64.9763) -> (-162.7837, -64.9763) centre (-169.5819, -64.5335) ccw
  spline S1 degree 2 poles (-154.9924, -57.4075) (-162.7837, -57.4075) (-162.7837, -64.9763) knots 0 0 0 1 1 1
  line L837 (-154.9924, -57.4075) -> (-35.7006, -57.4075)
  spline S2 degree 2 poles (-35.7006, -57.4075) (-27.9093, -57.4075) (-27.9093, -64.9763) knots 0 0 0 1 1 1
  arc A1 (-27.9093, -64.9763) -> (-14.3129, -64.9763) centre (-21.1111, -64.5335) ccw
  spline S3 degree 2 poles (-6.5216, -57.4075) (-14.3129, -57.4075) (-14.3129, -64.9763) knots 0 0 0 1 1 1
  line L838 (-167.2132, -68.8727) -> (-171.8315, -68.9414)
  line L839 (-171.8315, -68.9414) -> (-174.2002, -64.9763)
  line L840 (-174.2002, -64.9763) -> (-171.9506, -60.9423)
  line L841 (-171.9506, -60.9423) -> (-167.3323, -60.8736)
  line L842 (-167.3323, -60.8736) -> (-164.9636, -64.8387)
  line L843 (-164.9636, -64.8387) -> (-167.2132, -68.8727)
  line L844 (-18.8615, -68.9414) -> (-23.4798, -68.8727)
  line L845 (-23.4798, -68.8727) -> (-25.7294, -64.8387)
  line L846 (-25.7294, -64.8387) -> (-23.3607, -60.8736)
  line L847 (-23.3607, -60.8736) -> (-18.7424, -60.9423)
  line L848 (-18.7424, -60.9423) -> (-16.4928, -64.9763)
  line L849 (-16.4928, -64.9763) -> (-18.8615, -68.9414)
  spline S4 degree 2 poles (-23.4739, -0.2575) (-31.3819, -0.2565) (-31.3817, 7.3119) knots 0 0 0 1 1 1
  arc A2 (-31.3817, 7.3119) -> (-44.977, 7.3123) centre (-38.1793, 6.8699) ccw
  spline S5 degree 2 poles (-52.8852, -0.2567) (-44.9772, -0.2561) (-44.977, 7.3123) knots 0 0 0 1 1 1
  line L850 (-52.8852, -0.2567) -> (-52.887, -0.2573)
  line L851 (-52.887, -0.2573) -> (-137.8078, -0.2567)
  spline S6 degree 2 poles (-137.8078, -0.2567) (-145.7158, -0.2561) (-145.716, 7.3123) knots 0 0 0 1 1 1
  arc A3 (-145.716, 7.3123) -> (-159.3113, 7.3119) centre (-152.5137, 6.8699) ccw
  spline S7 degree 2 poles (-167.0351, -0.2565) (-159.3111, -0.1679) (-159.3113, 7.3119) knots 0.011703 0.011703 0.011703 1 1 1
  line L852 (-167.0351, -0.2565) -> (-188.597, -0.2563)
  line L853 (-154.7632, 3.2095) -> (-157.132, 7.1747)
  line L854 (-157.132, 7.1747) -> (-154.8824, 11.2086)
  line L855 (-154.8824, 11.2086) -> (-150.2641, 11.2774)
  line L856 (-150.2641, 11.2774) -> (-147.8954, 7.3122)
  line L857 (-147.8954, 7.3122) -> (-150.145, 3.2783)
  line L858 (-150.145, 3.2783) -> (-154.7632, 3.2095)
  line L859 (-35.9298, 3.2095) -> (-40.548, 3.2783)
  line L860 (-40.548, 3.2783) -> (-42.7976, 7.3122)
  line L861 (-42.7976, 7.3122) -> (-40.4289, 11.2774)
  line L862 (-40.4289, 11.2774) -> (-35.8106, 11.2086)
  line L863 (-35.8106, 11.2086) -> (-33.561, 7.1747)
  line L864 (-33.561, 7.1747) -> (-35.9298, 3.2095)
  dimension "d21" = 1
  dimension "d22" = 1
  dimension "d23" = 1
  dimension "d24" = 1
  dimension "d25" = 1
  dimension "d26" = 1
  constraint perpendicular L685 L686
  constraint parallel L685 L687
  constraint parallel L686 L688
  constraint coincident L327.end L328.start
  constraint perpendicular L328 L685
  constraint coincident L503.end L504.start
  constraint perpendicular L689 L690
  constraint parallel L689 L691
  constraint parallel L690 L692
  constraint coincident L514.end L515.start
  constraint perpendicular L515 L689